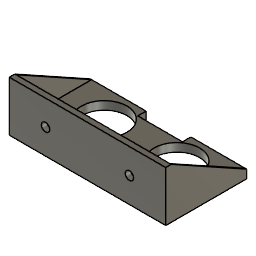
Mount (Autodesk Fusion 360 design; units mm, degrees)
Autodesk Fusion 360 part; units mm, degrees
sketch "Sketch1" plane through (0, 0, 0) normal (0, 0, 1) x (1, 0, 0)
  line L0 (27.5, -10) -> (-27.5, -10)
  line L1 (-27.5, -10) -> (-27.5, 10)
  line L2 (-27.5, 10) -> (27.5, 10)
  line L3 (27.5, 10) -> (27.5, -10)
  line L4 (27.5, -10) -> (-27.5, 10) construction
  line L5 (-27.5, -10) -> (27.5, 10) construction
  line L6 (0, 0) -> (13, 0) construction
  line L7 (0, 0) -> (-13, 0) construction
  circle A0 centre (13, 0) radius 8.125
  circle A1 centre (-13, 0) radius 8.125
  line L8 (-27.5, -10) -> (27.5, -10)
  line L9 (27.5, -10) -> (27.5, -17)
  line L10 (27.5, -17) -> (-27.5, -17)
  line L11 (-27.5, -17) -> (-27.5, -10)
  line L12 (0, 10) -> (-8, 10)
  line L13 (-8, 10) -> (8, 10)
  line L14 (8, 10) -> (8, 7)
  line L15 (8, 7) -> (-8, 7)
  line L16 (-8, 7) -> (-8, 10)
  line L17 (-7, -5.75) -> (7, -5.75)
  line L18 (7, -5.75) -> (7, -14.25)
  line L19 (7, -14.25) -> (-7, -14.25)
  line L20 (-7, -14.25) -> (-7, -5.75)
  line L21 (-7, -5.75) -> (7, -14.25) construction
  line L22 (7, -5.75) -> (-7, -14.25) construction
  point P0 (0, -10)
  dimension "d1" = 55
  dimension "d2" = 20
  dimension "d3" = 13
  dimension "d4" = 13
  dimension "d5" = 16.25
  dimension "d6" = 16.25
  dimension "d7" = 7
  dimension "d8" = 8
  dimension "d9" = 16
  dimension "d10" = 3
  dimension "d11" = 14
  dimension "d12" = 8.5
  constraint horizontal L0
  constraint perpendicular L0 L1
  constraint parallel L0 L2
  constraint parallel L1 L3
  constraint coincident L4 L6.start
  constraint coincident L5 L6.start
  constraint coincident L6.start L7.start
  constraint horizontal L6
  constraint parallel L6 L7
  constraint coincident L6.end A0.centre
  constraint coincident L7.end A1.centre
  constraint horizontal L8
  constraint vertical L9
  constraint horizontal L10
  constraint vertical L11
  constraint midpoint L2 L12.start
  constraint parallel L2 L12
  constraint horizontal L13
  constraint vertical L14
  constraint horizontal L15
  constraint vertical L16
  constraint horizontal L17
  constraint perpendicular L17 L18
  constraint parallel L17 L19
  constraint parallel L18 L20
  constraint coincident L21 P0
  constraint coincident L22 P0
  constraint midpoint L0 P0
  measures "d1" distance of L1.end L2.end
  measures "d2" distance of L0.end L1.end
  measures "d3" distance of L6.start L6.end
  measures "d4" distance of L6.start L7.end
  measures "d5" diameter of A0
  measures "d6" diameter of A1
  measures "d7" distance of L0.end L10.end
  measures "d8" distance of L12.start L12.end
  measures "d9" distance of L12.end L13.end
  measures "d10" distance of L12.end L15.end
  measures "d11" distance of L18.end L19.end
  measures "d12" distance of L17.end L18.end
extrude "Extrude1" add sketch "Sketch1" along normal blind 3 contours L0 L8 L9 L10 L11 L18 L19 L20 | L0 L1 L2 L3 L8 L14 L15 L16 L17 L18 L20
sketch "Sketch2" plane through (0, -17, 0) normal (0, -1, 0) x (1, 0, 0)
  line L0 (-27.5, 0) -> (27.5, 0)
  line L1 (27.5, 0) -> (27.5, 3)
  line L2 (27.5, 3) -> (-27.5, 3)
  line L3 (-27.5, 3) -> (-27.5, 0)
  line L4 (-27.5, 0) -> (27.5, 0)
  line L5 (27.5, 0) -> (27.5, 18)
  line L6 (27.5, 18) -> (-27.5, 18)
  line L7 (-27.5, 18) -> (-27.5, 0)
  line L8 (-27.5, 18) -> (27.5, 0) construction
  line L9 (-27.5, 0) -> (27.5, 18) construction
  line L10 (0, 9) -> (15, 9) construction
  line L11 (0, 9) -> (-15, 9) construction
  circle A0 centre (15, 9) radius 1.5
  circle A1 centre (-15, 9) radius 1.5
  dimension "d15" = 55
  dimension "d16" = 18
  dimension "d17" = 15
  dimension "d18" = 15
  dimension "d19" = 3
  dimension "d20" = 3
  constraint horizontal L4
  constraint vertical L5
  constraint horizontal L6
  constraint vertical L7
  constraint coincident L0.start L3.end
  constraint coincident L0.end L1.start
  constraint midpoint L8 L10.start
  constraint perpendicular L5 L10
  constraint parallel L10 L11
  constraint coincident L10.end A0.centre
  constraint coincident L11.end A1.centre
  measures "d15" distance of L0.start L0.end
  measures "d16" distance of L0.start L6.end
  measures "d17" distance of L10.start L10.end
  measures "d18" distance of L10.start L11.end
  measures "d19" diameter of A0
  measures "d20" diameter of A1
extrude "Extrude2" add sketch "Sketch2" along normal blind 2
sketch "Sketch3" plane through (-27.5, 0, 0) normal (-1, 0, 0) x (0, -1, 0)
  line L0 (-10, 0) -> (19, 0)
  line L1 (19, 0) -> (19, 18)
  line L2 (19, 18) -> (17, 18)
  line L3 (17, 18) -> (17, 3)
  line L4 (17, 3) -> (-10, 3)
  line L5 (-10, 3) -> (-10, 0)
  line L6 (17, 18) -> (-10, 3)
  constraint coincident L2.end L3.start
  constraint coincident L4.end L5.start
extrude "Extrude3" add sketch "Sketch3" along normal blind 0.5
sketch "Sketch4" plane through (27.5, 0, 0) normal (1, 0, 0) x (0, 1, 0)
  line L0 (-19, 0) -> (10, 0)
  line L1 (10, 0) -> (10, 3)
  line L2 (10, 3) -> (-17, 3)
  line L3 (-17, 3) -> (-17, 18)
  line L4 (-17, 18) -> (-19, 18)
  line L5 (-19, 18) -> (-19, 0)
  line L6 (-17, 18) -> (10, 3)
  constraint coincident L3.end L4.start
  constraint coincident L1.end L2.start
extrude "Extrude4" add sketch "Sketch4" along normal blind 0.5
